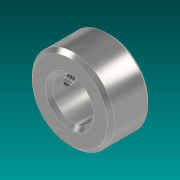
# Autodesk Inventor part: askraag 8mm
Saved by Autodesk Inventor 2020.2 (Build 242310000, 310)
## iProperties
Created: 2020-05-15
Part Number: askraag 8mm
Material: Stainless Steel
Document SubType Name: Modeling
Designer: Svend
Density: 8 g/cm^3
Appearance: Semi-Polished
Author: Svend
Autodesk Inventor part; units mm, degrees
ref_plane "YZ Plane" through (0, 0, 0) normal (1, 0, 0) x (0, 1, 0)
ref_plane "XZ Plane" through (0, 0, 0) normal (0, 1, 0) x (-1, 0, 0)
ref_plane "XY Plane" through (0, 0, 0) normal (0, 0, 1) x (1, 0, 0)
sketch "Sketch1" plane through (0, 0, 0) normal (0, 0, 1) x (1, 0, 0)
  circle A0 centre (0, 0) radius 8
  circle A1 centre (0, 0) radius 4
  dimension "d0" = 16
  dimension "d1" = 8
  constraints: 2 centre point, 2 coincident
  measures "d0" diameter of A0
  measures "d1" diameter of A1
extrude "Extrusion1" add sketch "Sketch1" along normal blind 7.9
chamfer "Chamfer1" distance 0.7 angle 45 4 edges at (-8, 0, 0) (-8, 0, 7.9) (-4, 0, 0) (-4, 0, 7.9)
sketch "Sketch2" plane through (0, 0, 0) normal (1, 0, 0) x (0, 1, 0)
  line L0 (-4.7, 0) -> (4.7, 0) projected
  line L1 (4.7, 7.9) -> (-4.7, 7.9) projected
  point P0 (0, 0)
  point P1 (0, 3.95)
  point P2 (0, 0)
  dimension "d7" = 3.95
  constraints: 1 midpoint, 1 vertical alignment
  measures "d7" distance of point (0, 0) point (0, 3.95)
hole "Hole1" at (0, 0, 3.95) direction (-1, 0, 0) diameter 2.459 end through all thread size "M3x0.5" class "6H" standard "ISO Metric profile"
chamfer "Chamfer2" distance 0.5 angle 45 1 edges at (-8, 0.0002, 5.1795)
body "Solid1"
